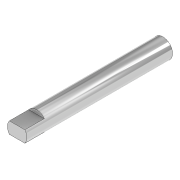
# Autodesk Inventor part: 5x37.5mm Rod
Saved by Autodesk Inventor 2020 (Build 240168000, 168)
## iProperties
Created: 2021-06-26
Part Number: 5x37.5mm Rod
Material: Generic
Document SubType Name: Modeling
Designer: Coy
Density: 1 g/cm^3
Appearance: Chrome - Polished
Author: Coy
Autodesk Inventor part; units mm, degrees
ref_plane "YZ Plane" through (0, 0, 0) normal (1, 0, 0) x (0, 1, 0)
ref_plane "XZ Plane" through (0, 0, 0) normal (0, 1, 0) x (-1, 0, 0)
ref_plane "XY Plane" through (0, 0, 0) normal (0, 0, 1) x (1, 0, 0)
sketch "Sketch1" plane through (0, 0, 0) normal (0, 0, 1) x (1, 0, 0)
  circle A0 centre (0, 0) radius 2.5
  dimension "d0" = 5
  constraints: 1 centre point, 1 coincident
  measures "d0" diameter of A0
extrude "Extrusion1" add sketch "Sketch1" against normal blind 37.5
sketch "Sketch2" plane through (0, 0, 0) normal (0, 0, 1) x (1, 0, 0)
  line L0 (-9.2586, 1.5) -> (11.2759, 1.5)
  line L1 (11.2759, -1.5) -> (-9.2586, -1.5)
  circle A0 centre (0, 0) radius 2.5 projected
  point P0 (2, 1.5)
  point P1 (-2, 1.5)
  point P2 (-2, -1.5)
  point P3 (2, -1.5)
  dimension "d3" = 3
  dimension "d4" = 1.5
  constraints: 4 end point, 2 horizontal
  measures "d3" distance between parallel lines of L0 L1
  measures "d4" distance from line of point (0, 0) L0
extrude "Extrusion2" cut sketch "Sketch2" against normal blind 5 contours A0 L0 | L1 A0
equation "\"d4\" = 0.5 * d3"
body "Solid1"
